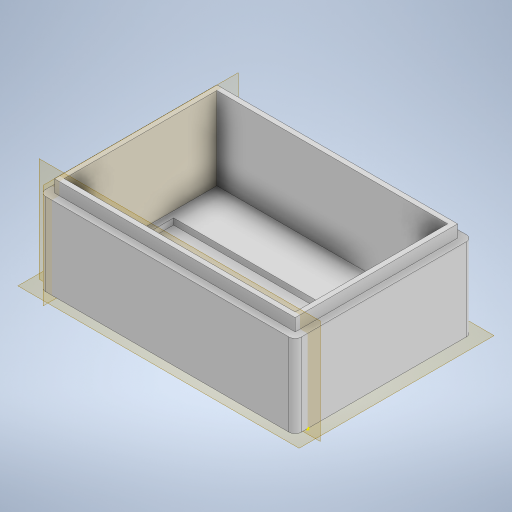
# Autodesk Inventor part: ieee_box
Saved by Autodesk Inventor 2024 (Build 280153000, 153)
## iProperties
Created: 2023-11-20
Part Number: ieee_box
Material: Generic
Document SubType Name: Modeling
Designer: sophi
Density: 1 g/cm^3
Appearance: Default
Author: sophi
Autodesk Inventor part; units mm, degrees
sketch "Sketch1" plane through (0, 0, 0) normal (0, 1, 0) x (-1, 0, 0)
  line L0 (0, 0) -> (-56, 0)
  line L1 (-56, 0) -> (-56, -37)
  line L2 (-56, -37) -> (0, -37)
  line L3 (0, -37) -> (0, 0)
  line L4 (3, -40) -> (-59, -40)
  line L5 (-59, -40) -> (-59, 3)
  line L6 (-59, 3) -> (3, 3)
  line L7 (3, 3) -> (3, -40)
  dimension "d0" = 56
  dimension "d1" = 37
  dimension "d2" = 3
  constraints: 16 end point, 4 parallel, 2 perpendicular, 1 horizontal, 3 other
  measures "d0" distance of L1.end L2.end
  measures "d1" distance of L0.end L1.end
  measures "d2" distance between parallel lines of L4 L2
extrude "Extrusion1" add sketch "Sketch1" along normal blind 3 contours L3 L2 L1 L0 | L4 L5 L6 L7
sketch "Sketch2" plane through (0, 3, 0) normal (0, 1, 0) x (1, 0, 0)
  line L0 (-3, -3) -> (59, -3) projected
  line L1 (59, -3) -> (59, 40) projected
  line L2 (-3, -3) -> (59, -3)
  line L3 (59, -3) -> (59, 40)
  line L4 (59, 40) -> (-3, 40)
  line L5 (-3, 40) -> (-3, -3)
  line L6 (0, 37) -> (56, 37)
  line L7 (56, 37) -> (56, 0)
  line L8 (56, 0) -> (0, 0)
  line L9 (0, 0) -> (0, 37)
  point P0 (0, 0)
  dimension "d5" = 3
  constraints: 16 end point, 4 parallel, 2 perpendicular, 1 horizontal, 3 other
  measures "d5" distance between parallel lines of L4 L6
extrude "Extrusion2" add sketch "Sketch2" along normal blind 20
sketch "Sketch3" plane through (0, 3, 0) normal (0, 1, 0) x (1, 0, 0)
  line L0 (1.5, 25) -> (54.5, 25)
  line L1 (54.5, 25) -> (54.5, 0)
  line L2 (54.5, 0) -> (1.5, 0)
  line L3 (1.5, 0) -> (1.5, 25)
  line L4 (0, 37) -> (56, 37) projected
  line L5 (71.4, 0) -> (-15.4, 0) projected
  point P0 (0, 0)
  point P1 (28, 37)
  point P2 (28, 25)
  dimension "d8" = 53
  dimension "d9" = 25
  dimension "d10" = 0
  dimension "d12" = 0
  constraints: 8 end point, 2 midpoint, 2 parallel, 1 horizontal, 1 perpendicular
  measures "d8" distance of L0.start L0.end
  measures "d9" distance of L2.end L0.start
  measures "d10" horizontal distance of point (28, 37) point (28, 25)
  measures "d12" distance between parallel lines of L5 L2
extrude "Extrusion3" cut sketch "Sketch3" against normal blind 1.5
sketch "Sketch4" plane through (0, 23, 0) normal (0, 1, 0) x (1, 0, 0)
  line L0 (-3, -3) -> (59, -3) projected
  line L1 (59, -3) -> (59, 40) projected
  line L2 (-3, -3) -> (59, -3)
  line L3 (59, -3) -> (59, 40)
  line L4 (59, 40) -> (-3, 40)
  line L5 (-3, 40) -> (-3, -3)
  line L6 (-1.2, 38.2) -> (57.2, 38.2)
  line L7 (57.2, 38.2) -> (57.2, -1.2)
  line L8 (57.2, -1.2) -> (-1.2, -1.2)
  line L9 (-1.2, -1.2) -> (-1.2, 38.2)
  point P0 (0, 0)
  dimension "d15" = 1.8
  constraints: 16 end point, 4 parallel, 2 perpendicular, 1 horizontal, 3 other
  measures "d15" distance between parallel lines of L4 L6
extrude "Extrusion4" cut sketch "Sketch4" against normal blind 3
fillet "Fillet1" radius 1.5 4 edges at (-3, 10, 3) (59, 10, 3) (59, 10, -40) (-3, 10, -40)
sketch "Sketch5" plane through (59, 0, 1.5) normal (1, 0, 0) x (0, 0, -1)
  point P0 (1.5, 0)
equation "\"d0\" = length_inner"
equation "\"d1\" = width_inner"
equation "\"d2\" = thickness"
equation "\"d3\" = thickness"
equation "\"d5\" = thickness"
equation "\"d6\" = height_inner"
equation "\"d8\" = length_batt"
equation "\"d9\" = width_batt"
equation "\"d13\" = 0.5 * thickness"
equation "\"d15\" = 0.6 * thickness"
equation "\"d16\" = thickness"
equation "\"d18\" = 0.5 * thickness"
equation "\"length_inner\" = 56"
equation "\"width_inner\" = 37"
equation "\"height_inner\" = 20"
equation "\"thickness\" = 3"
equation "\"length_batt\" = 53"
equation "\"width_batt\" = 25"
body "Solid1"
